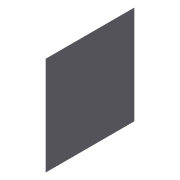
# Autodesk Inventor part: side350x390
Saved by Autodesk Inventor 2014 SP1 (Build 180222100, 222)
## iProperties
Created: 2015-02-11
Part Number: side350x390
Material: Generic
Document SubType Name: Modeling
Designer: Simen
Density: 1 g/cm^3
Appearance: Default
Author: Simen
Autodesk Inventor part; units mm, degrees
ref_plane "YZ Plane" through (0, 0, 0) normal (1, 0, 0) x (0, 1, 0)
ref_plane "XZ Plane" through (0, 0, 0) normal (0, 1, 0) x (-1, 0, 0)
ref_plane "XY Plane" through (0, 0, 0) normal (0, 0, 1) x (1, 0, 0)
sketch "Sketch1" plane through (0, 0, 0) normal (1, 0, 0) x (0, 1, 0)
  line L0 (-65.6817, 34.7306) -> (284.3183, 34.7306)
  line L1 (284.3183, 34.7306) -> (284.3183, -355.2694)
  line L2 (284.3183, -355.2694) -> (-65.6817, -355.2694)
  line L3 (-65.6817, -355.2694) -> (-65.6817, 34.7306)
  point P0 (0, 0)
  dimension "d0" = 350
  dimension "d1" = 390
  constraints: 8 end point, 2 parallel, 1 horizontal, 1 perpendicular
  measures "d0" distance of L1.end L2.end
  measures "d1" distance of L0.end L1.end
extrude "Extrusion1" add sketch "Sketch1" along normal blind 0.8
body "Solid1"
